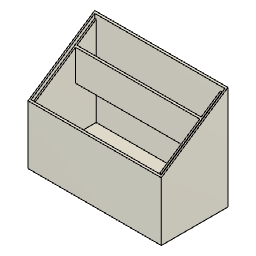
exterior v4 (Autodesk Fusion 360 design; units mm, degrees)
Autodesk Fusion 360 part; units mm, degrees
note: some values were not read from the file. Set by a fixed rule: which face or edge a step refers to.
sketch "Sketch1" plane through (0, 0, 0) normal (1, 0, 0) x (0, 0, -1)
  line L0 (0, 0) -> (0, 70)
  line L1 (0, 70) -> (-45, 39.6471)
  line L2 (0, 70) -> (-53, 70) construction
  line L3 (0, 0) -> (-45, 0)
  line L4 (-45, 0) -> (-45, 39.6471)
  dimension "d1" = 70
  dimension "d2" = 34
  constraint coincident L0.start L3.start
  constraint vertical L0
  constraint horizontal L2
  constraint perpendicular L0 L3
  constraint perpendicular L3 L4
  measures "d1" distance of L0.start L0.end
  measures "d2" angle of L1 L2
extrude "Extrude1" add sketch "Sketch1" along normal blind 90 makes body 1
shell "Shell1" thickness 1 removed faces 1 at (30, 59.8824, 15) on bodies 1
extrude "Extrude2" cut 1 faces at (30.3333, 1, 15.3333) along direction (0, -1, 0) blind 20 on bodies 1 bodies 1
ref_plane "WorkPlane1" through (2, 34.6627, 22.5) normal (1, 0, 0) x (0, 0, -1)
sketch "Sketch4" plane through (2, 34.6627, 22.5) normal (1, 0, 0) x (0, 0, -1)
  line L0 (21.5, -34.6627) -> (21.5, 34.6627)
  line L1 (21.5, 34.6627) -> (-21.5, 5.6589)
  line L2 (-21.5, 5.6589) -> (-21.5, -34.6627)
  line L3 (-21.5, -34.6627) -> (21.5, -34.6627)
  line L4 (-20.5, -33.6627) -> (20.5, -33.6627)
  line L5 (20.5, -33.6627) -> (20.5, 32.782)
  line L6 (20.5, 32.782) -> (-20.5, 5.1272)
  line L7 (-20.5, 5.1272) -> (-20.5, -33.6627)
  line L8 (-20.5, -33.6627) -> (20.5, -33.6627)
  line L9 (20.5, -33.6627) -> (20.5, -28.6627)
  line L10 (20.5, -28.6627) -> (-20.5, -28.6627)
  line L11 (-20.5, -28.6627) -> (-20.5, -33.6627)
  dimension "d16" = -1
  dimension "d17" = 5
  constraint horizontal L8
  constraint vertical L9
  constraint horizontal L10
  constraint vertical L11
  measures "d17" distance of L4.start L10.end
extrude "Extrude5" add sketch "Sketch4" along normal blind 1 separate body contours L5 L6 L7 L10 makes body 2
copy_body "CopyPasteBodies1" bodies 2 makes body 3
move_body "Move1" bodies 3 to x (1, 0, 0) y (0, 1, 0) z (0, 0, 1) at (85, 0, 0)
sketch "Sketch5" plane through (0, 6, 0) normal (0, -1, 0) x (1, 0, 0)
  line L0 (87, 43) -> (87, 2)
  line L1 (87, 2) -> (88, 2)
  line L2 (88, 2) -> (88, 43)
  line L3 (88, 43) -> (87, 43)
  line L4 (87, 43) -> (3, 43)
  line L5 (3, 43) -> (3, 2)
  line L6 (3, 2) -> (87, 2)
  line L7 (87, 2) -> (87, 43)
  constraint horizontal L4
  constraint vertical L5
  constraint horizontal L6
  constraint vertical L7
  constraint coincident L0.start L3.end
extrude "Extrude6" add sketch "Sketch5" against normal blind 1 contours L0 L4 L5 L6 L7 bodies 2 3
sketch "Sketch6" plane through (0, 7, 0) normal (0, 1, 0) x (-1, 0, 0)
  line L0 (-87, 43) -> (-87, 2)
  line L1 (-87, 2) -> (-3, 2)
  line L2 (-3, 2) -> (-3, 43)
  line L3 (-3, 43) -> (-87, 43)
  line L4 (-3, 15) -> (-87, 15)
  line L5 (-87, 15) -> (-87, 16)
  line L6 (-87, 16) -> (-3, 16)
  line L7 (-3, 16) -> (-3, 15)
  dimension "d22" = 1
  constraint horizontal L4
  constraint vertical L5
  constraint horizontal L6
  constraint vertical L7
  constraint coincident L0 L5.end
  constraint coincident L2 L4.start
  measures "d22" distance of L4.start L6.end
extrude "Extrude7" add sketch "Sketch6" along normal blind 55 contours L0 L2 L4 L5 L6 L7 bodies 2
extrude "Extrude8" cut 1 faces at (3, 59.5593, 15.6667) along direction (1, 0, 0) blind 85 on bodies 2 bodies 2
sketch "Sketch7" plane through (0, 0, 16) normal (0, 0, 1) x (1, 0, 0)
  line L0 (87, 58.0016) -> (3, 58.0016)
  line L1 (3, 58.0016) -> (3, 7)
  line L2 (3, 7) -> (87, 7)
  line L3 (87, 7) -> (87, 58.0016)
  line L4 (87, 7) -> (3, 7)
  line L5 (3, 7) -> (3, 37)
  line L6 (3, 37) -> (87, 37)
  line L7 (87, 37) -> (87, 7)
  dimension "d27" = 84
  dimension "d28" = 30
  constraint horizontal L4
  constraint vertical L5
  constraint horizontal L6
  constraint vertical L7
  constraint coincident L2.end L3.start
  measures "d27" distance of L2.end L1.end
  measures "d28" distance of L2.end L6.end
extrude "Extrude9" cut sketch "Sketch7" against normal blind 5 contours L1 L2 L3 L4 L5 L6 L7 bodies 2
